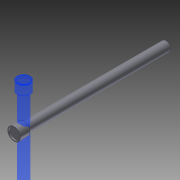
# Autodesk Inventor part: Pusher.Pushrod
Saved by Autodesk Inventor 2011 (Build 150239000, 239)
## iProperties
Created: 2011-04-01
Part Number: Pusher.Pushrod
Material: Stainless Steel
Document SubType Name: Sheet Metal
Designer: Rob
Density: 8.08 g/cm^3
Sheet Metal Rule: Default_mm
Mass: 22.4357 g
Surface Area: 19.4904 cm^2
Volume: 2.7767 cm^3
Author: Rob
Autodesk Inventor part; units mm, degrees
ref_plane "YZ Plane" through (0, 0, 0) normal (1, 0, 0) x (0, 1, 0)
ref_plane "XZ Plane" through (0, 0, 0) normal (0, 1, 0) x (-1, 0, 0)
ref_plane "XY Plane" through (0, 0, 0) normal (0, 0, 1) x (1, 0, 0)
sketch "Sketch1" plane through (0, 0, 0) normal (0, 0, 1) x (1, 0, 0)
  line L0 (-3, 0) -> (-3, 88.9)
  line L1 (-3, 88.9) -> (0, 88.9)
  line L2 (0, 88.9) -> (0, 0)
  line L3 (-3, 0) -> (-4, 0)
  line L4 (-4, 0) -> (-4, -6)
  line L5 (-4, -6) -> (-3.5, -6)
  line L6 (-3.5, -6) -> (-3.5, -5)
  line L7 (-3.5, -5) -> (0, -5)
  line L8 (0, -5) -> (0, 0)
  dimension "d0" = 3
  dimension "d1" = 88.9
  dimension "d7" = 6
  dimension "d9" = 4
  dimension "d10" = 1
  dimension "d11" = 0.5
  constraints: 18 end point, 3 horizontal, 3 parallel, 2 vertical, 1 perpendicular, 1 point on line
  measures "d0" distance of L0.end L1.end
  measures "d1" distance of L0.start L0.end
  measures "d7" distance of L3.end L4.end
  measures "d9" distance between parallel lines of L2 L4
  measures "d10" distance of L5.end L6.end
  measures "d11" distance of L4.end L5.end
revolve "Revolution1" add sketch "Sketch1" angle 360 about axis through (0, 88.9, 0) along (0, -1, 0)
equation "\"BendRadius\" = Thickness"
equation "\"BendReliefWidth\" = Thickness"
equation "\"BendReliefDepth\" = 0.5 * Thickness"
equation "\"CornerReliefSize\" = 4 * Thickness"
equation "\"MinimumRemnant\" = 2 * Thickness"
equation "\"TransitionRadius\" = BendRadius"
equation "\"JacobiRadiusSize\" = BendRadius"
equation "\"GapSize\" = Thickness"
equation "\"Thickness\" = 0.5"
body "Solid1"
